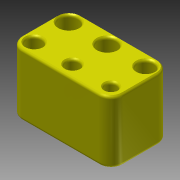
# Autodesk Inventor part: Porta destornilladores
Saved by Autodesk Inventor 2014 (Build 180170000, 170)
## iProperties
Created: 2017-01-13
Part Number: Porta destornilladores
Material: Generic
Document SubType Name: Modeling
Designer: Rubén
Density: 1 g/cm^3
Appearance: Smooth - Yellow
Author: Rubén
Autodesk Inventor part; units mm, degrees
ref_plane "YZ Plane" through (0, 0, 0) normal (1, 0, 0) x (0, 1, 0)
ref_plane "XZ Plane" through (0, 0, 0) normal (0, 1, 0) x (-1, 0, 0)
ref_plane "XY Plane" through (0, 0, 0) normal (0, 0, 1) x (1, 0, 0)
sketch "Sketch1" plane through (0, 0, 0) normal (0, 1, 0) x (-1, 0, 0)
  circle A0 centre (12.3553, -5.5714) radius 2.95
  circle A1 centre (0, -5.5714) radius 2.9
  circle A2 centre (-12.3553, -5.5714) radius 2.6
  circle A3 centre (12.3553, 5.5714) radius 2.425
  circle A4 centre (0, 5.5714) radius 2.1
  circle A5 centre (-12.3553, 5.5714) radius 1.8
  line L0 (15.4441, -10.9214) -> (9.2665, -10.9214) construction
  line L1 (9.2665, -10.9214) -> (6.1776, -5.5714) construction
  line L2 (6.1776, -5.5714) -> (9.2665, -0.2214) construction
  line L3 (9.2665, -0.2214) -> (15.4441, -0.2214) construction
  line L4 (15.4441, -0.2214) -> (18.5329, -5.5714) construction
  line L5 (18.5329, -5.5714) -> (15.4441, -10.9214) construction
  circle A6 centre (12.3553, -5.5714) radius 6.1776 construction
  line L6 (-10.3346, 2.0714) -> (-14.376, 2.0714) construction
  line L7 (-14.376, 2.0714) -> (-16.3967, 5.5714) construction
  line L8 (-16.3967, 5.5714) -> (-14.376, 9.0714) construction
  line L9 (-14.376, 9.0714) -> (-10.3346, 9.0714) construction
  line L10 (-10.3346, 9.0714) -> (-8.3138, 5.5714) construction
  line L11 (-8.3138, 5.5714) -> (-10.3346, 2.0714) construction
  line L12 (-3.0888, -10.9214) -> (-6.1776, -5.5714) construction
  line L13 (-6.1776, -5.5714) -> (-3.0888, -0.2214) construction
  line L14 (-3.0888, -0.2214) -> (3.0888, -0.2214) construction
  line L15 (3.0888, -0.2214) -> (6.1776, -5.5714) construction
  line L16 (6.1776, -5.5714) -> (3.0888, -10.9214) construction
  line L17 (3.0888, -10.9214) -> (-3.0888, -10.9214) construction
  line L18 (-17.9845, -5.5714) -> (-15.1699, -0.6964) construction
  line L19 (-15.1699, -0.6964) -> (-9.5407, -0.6964) construction
  line L20 (-9.5407, -0.6964) -> (-6.7261, -5.5714) construction
  line L21 (-6.7261, -5.5714) -> (-9.5407, -10.4464) construction
  line L22 (-9.5407, -10.4464) -> (-15.1699, -10.4464) construction
  line L23 (-15.1699, -10.4464) -> (-17.9845, -5.5714) construction
  line L24 (14.8379, 9.8714) -> (17.3205, 5.5714) construction
  line L25 (17.3205, 5.5714) -> (14.8379, 1.2714) construction
  line L26 (14.8379, 1.2714) -> (9.8727, 1.2714) construction
  line L27 (9.8727, 1.2714) -> (7.3901, 5.5714) construction
  line L28 (7.3901, 5.5714) -> (9.8727, 9.8714) construction
  line L29 (9.8727, 9.8714) -> (14.8379, 9.8714) construction
  line L30 (2.2517, 9.4714) -> (4.5033, 5.5714) construction
  line L31 (4.5033, 5.5714) -> (2.2517, 1.6714) construction
  line L32 (2.2517, 1.6714) -> (-2.2517, 1.6714) construction
  line L33 (-2.2517, 1.6714) -> (-4.5033, 5.5714) construction
  line L34 (-4.5033, 5.5714) -> (-2.2517, 9.4714) construction
  line L35 (-2.2517, 9.4714) -> (2.2517, 9.4714) construction
  circle A7 centre (0, 5.5714) radius 4.5033 construction
  circle A8 centre (12.3553, 5.5714) radius 4.9652 construction
  circle A9 centre (-12.3553, -5.5714) radius 5.6292 construction
  circle A10 centre (0, -5.5714) radius 6.1776 construction
  circle A11 centre (-12.3553, 5.5714) radius 4.0415 construction
  line L36 (-12.3553, 5.5714) -> (0, 5.5714) construction
  line L37 (0, 5.5714) -> (12.3553, 5.5714) construction
  line L38 (12.3553, -5.5714) -> (0, -5.5714) construction
  line L39 (0, -5.5714) -> (-12.3553, -5.5714) construction
  line L40 (-12.3553, 9.5214) -> (12.3553, 9.5214)
  line L41 (12.3553, -9.5214) -> (-12.3553, -9.5214)
  line L42 (-16.3053, -5.5714) -> (-16.3053, 5.5714)
  line L43 (0, 5.5714) -> (0, 9.5214) construction
  line L44 (-12.3553, 0) -> (-16.3053, 0) construction
  line L45 (0, -5.5714) -> (0, -9.5214) construction
  line L46 (12.3553, 5.5714) -> (12.3553, -5.5714) construction
  line L47 (-12.3553, 5.5714) -> (-12.3553, -5.5714) construction
  line L48 (12.3553, 0.6062) -> (16.3053, 0.6062) construction
  line L49 (16.3053, 5.5714) -> (16.3053, -5.5714)
  line L50 (0, 0) -> (-12.3553, 0) construction
  line L51 (0, 5.5714) -> (0, 0) construction
  line L52 (0, 0) -> (0, -5.5714) construction
  arc A12 (12.3553, -9.5214) -> (16.3053, -5.5714) centre (12.3553, -5.5714) ccw
  arc A13 (16.3053, 5.5714) -> (12.3553, 9.5214) centre (12.3553, 5.5714) ccw
  arc A14 (-12.3553, 9.5214) -> (-16.3053, 5.5714) centre (-12.3553, 5.5714) ccw
  arc A15 (-16.3053, -5.5714) -> (-12.3553, -9.5214) centre (-12.3553, -5.5714) ccw
  dimension "d0" = 5.9
  dimension "d1" = 10.7
  dimension "d2" = 5.8
  dimension "d3" = 10.7
  dimension "d4" = 5.2
  dimension "d5" = 9.75
  dimension "d6" = 4.85
  dimension "d7" = 8.6
  dimension "d8" = 4.2
  dimension "d9" = 7.8
  dimension "d10" = 3.6
  dimension "d11" = 7
  dimension "d18" = 1
  constraints: 106 end point, 13 coincident, 11 centre point, 10 point on circle, 9 parallel, 9 tangent, 5 horizontal, 5 vertical, 4 equal length, 4 midpoint, 3 equal radius, 3 perpendicular, 2 point on line, 1 collinear, 1 horizontal alignment, 91 other
  measures "d0" diameter of A0
  measures "d1" distance between parallel lines of L5 L2
  measures "d2" diameter of A1
  measures "d3" distance between parallel lines of L17 L14
  measures "d4" diameter of A2
  measures "d5" distance between parallel lines of L21 L18
  measures "d6" diameter of A3
  measures "d7" distance between parallel lines of L26 L29
  measures "d8" diameter of A4
  measures "d9" distance between parallel lines of L31 L34
  measures "d10" diameter of A5
  measures "d11" distance between parallel lines of L6 L9
  measures "d18" distance edge to line of A0 L41
extrude "Extrusion1" add sketch "Sketch1" along normal blind 20
chamfer "Chamfer1" distance 0.5 angle 45 28 edges at (-9.9303, 20, 5.5714) (-9.4053, 20, -5.5714) (2.9, 20, -5.5714) (2.1, 20, 5.5714) (14.1553, 20, 5.5714) (14.9553, 20, -5.5714) (-9.9303, 0, 5.5714) (-9.4053, 0, -5.5714) (2.1, 0, 5.5714) (2.9, 0, -5.5714) (14.1553, 0, 5.5714) (14.9553, 0, -5.5714) (0, 0, -9.5214) (15.1484, 0, -8.3645) (16.3053, 0, 0) (15.1484, 0, 8.3645) (0, 0, 9.5214) (-15.1484, 0, 8.3645) (-16.3053, 0, 0) (-15.1484, 0, -8.3645) (0, 20, -9.5214) (-15.1484, 20, -8.3645) (-16.3053, 20, 0) (-15.1484, 20, 8.3645) (0, 20, 9.5214) (15.1484, 20, 8.3645) (16.3053, 20, 0) (15.1484, 20, -8.3645)
fillet "Fillet1" radius 1 28 edges at (-15.1484, 19.5005, -8.3645) (-16.3053, 19.5005, 0) (-15.1484, 19.5005, 8.3645) (0, 19.5005, 9.5214) (15.1484, 19.5005, 8.3645) (16.3053, 19.5005, 0) (15.1484, 19.5005, -8.3645) (0, 19.5005, -9.5214) (0, 0.4995, -9.5214) (15.1484, 0.4995, -8.3645) (16.3053, 0.4995, 0) (15.1484, 0.4995, 8.3645) (0, 0.4995, 9.5214) (-15.1484, 0.4995, 8.3645) (-16.3053, 0.4995, 0) (-15.1484, 0.4995, -8.3645) (-9.4053, 0.4995, -5.5714) (-9.9303, 0.4995, 5.5714) (2.1, 0.4995, 5.5714) (2.9, 0.4995, -5.5714) (14.9553, 0.4995, -5.5714) (14.1553, 0.4995, 5.5714) (-9.4053, 19.5005, -5.5714) (-9.9303, 19.5005, 5.5714) (2.9, 19.5005, -5.5714) (2.1, 19.5005, 5.5714) (14.9553, 19.5005, -5.5714) (14.1553, 19.5005, 5.5714)
body "Solid1"
